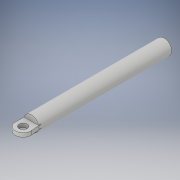
# Autodesk Inventor part: 圓柱3
Saved by Autodesk Inventor 2019 (Build 230136000, 136)
## iProperties
Created: 2021-03-25
Part Number: 圓柱3
Material: 一般
Document SubType Name: Modeling
Designer: cadlab
Density: 1 g/cm^3
Appearance: 預設
Author: cadlab
Autodesk Inventor part; units mm, degrees
ref_plane "YZ Plane" through (0, 0, 0) normal (1, 0, 0) x (0, 1, 0)
ref_plane "XZ Plane" through (0, 0, 0) normal (0, 1, 0) x (-1, 0, 0)
ref_plane "XY Plane" through (0, 0, 0) normal (0, 0, 1) x (1, 0, 0)
sketch "草圖1" plane through (0, 0, 0) normal (0, 0, 1) x (1, 0, 0)
  circle A0 centre (0, 0) radius 9.5
  dimension "d0" = 19
  constraints: 1 centre point, 1 coincident
  measures "d0" diameter of A0
extrude "擠出1" add sketch "草圖1" against normal blind 170
sketch "草圖2" plane through (0, 0, 0) normal (0, 1, 0) x (-1, 0, 0)
  line L0 (-9.5, 0) -> (9.5, 0) projected
  line L1 (9.5, 0) -> (9.5, 10.9087)
  line L2 (-10.4544, 9.9544) -> (-9.5, 0)
  arc A0 (9.5, 10.9087) -> (-10.4544, 9.9544) centre (-0.5, 10.9087) ccw
  circle A1 centre (-0.5, 10.9087) radius 5.099
  point P0 (0, 0)
  dimension "d3" = 10
  dimension "d4" = 10
  constraints: 4 end point, 2 centre point, 2 point on circle, 2 tangent, 1 coincident, 1 vertical
  measures "d3" distance of L2.start L0.start
  measures "d4" radius of A0
extrude "擠出2" add sketch "草圖2" along normal mid plane 5
delete faces "刪除面1" heal yes whole lump no faces at (9.3386, 2.2259, 0) (9.3386, -2.2259, 0) (-9.3386, 2.2259, 0) (-9.3386, -2.2259, 0)
